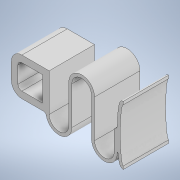
# Autodesk Inventor part: resortePlano0.8mm
Saved by Autodesk Inventor 2021.5 (Build 255421000, 421)
## iProperties
Created: 2024-11-30
Part Number: resortePlano0.8mm
Material: Genérico
Document SubType Name: Modeling
Designer: Joho_
Density: 1 g/cm^3
Appearance: Valor por defecto
Author: Joho_
## iProperties of the stored document _3DPrint.ipt
Created: 2024-11-30
Part Number: _3DPrint
Material: Genérico
Document SubType Name: Modeling
Designer: Joho_
Density: 1 g/cm^3
Appearance: Valor por defecto
Author: Joho_
Autodesk Inventor part; units mm, degrees
ref_plane "YZ Plane" through (0, 0, 0) normal (1, 0, 0) x (0, 1, 0)
ref_plane "XZ Plane" through (0, 0, 0) normal (0, 1, 0) x (-1, 0, 0)
ref_plane "XY Plane" through (0, 0, 0) normal (0, 0, 1) x (1, 0, 0)
sketch "Boceto1" plane through (0, 0, 0) normal (0, 0, 1) x (1, 0, 0)
  line L0 (3, -11.4) -> (3, -5.5)
  line L1 (3, -5.5) -> (-2.2, -5.5)
  arc A0 (-5.5, -2.2) -> (-2.2, -5.5) centre (-2.2, -2.2) ccw
  line L2 (-5.5, -2.2) -> (-5.5, 2.2)
  arc A1 (-2.2, 5.5) -> (-5.5, 2.2) centre (-2.2, 2.2) ccw
  line L3 (-2.2, 5.5) -> (3, 5.5)
  line L4 (3, 5.5) -> (3, 11.4)
  line L5 (3, 3) -> (-2.2, 3)
  arc A2 (-2.2, 3) -> (-3, 2.2) centre (-2.2, 2.2) ccw
  line L6 (-3, 2.2) -> (-3, -2.2)
  arc A3 (-3, -2.2) -> (-2.2, -3) centre (-2.2, -2.2) ccw
  line L7 (-2.2, -3) -> (3, -3)
  line L8 (3, -3) -> (3, 3)
  line L9 (-2.2, 3.25) -> (3.25, 3.25)
  line L10 (3.25, 3.25) -> (3.25, -3.25)
  line L11 (3.25, -3.25) -> (-2.2, -3.25)
  arc A4 (-3.25, -2.2) -> (-2.2, -3.25) centre (-2.2, -2.2) ccw
  line L12 (-3.25, -2.2) -> (-3.25, 2.2)
  arc A5 (-2.2, 3.25) -> (-3.25, 2.2) centre (-2.2, 2.2) ccw
  line L13 (-2.2, 5) -> (5, 5)
  line L14 (5, 5) -> (5, -5)
  line L15 (5, -5) -> (-2.2, -5)
  arc A6 (-5, -2.2) -> (-2.2, -5) centre (-2.2, -2.2) ccw
  line L16 (-5, -2.2) -> (-5, 2.2)
  arc A7 (-2.2, 5) -> (-5, 2.2) centre (-2.2, 2.2) ccw
  line L17 (22.2, 0) -> (23, 0)
  line L18 (10.2, 5) -> (11, 5)
  line L19 (11, 5) -> (11, -5)
  line L20 (11, -5) -> (10.2, -5)
  line L21 (10.2, -5) -> (10.2, 5)
  line L22 (16.2, 5) -> (17, 5)
  line L23 (17, 5) -> (17, -5)
  line L24 (17, -5) -> (16.2, -5)
  line L25 (16.2, -5) -> (16.2, 5)
  line L26 (22.2, 5) -> (23, 5)
  line L27 (23, 0) -> (23, -5)
  line L28 (23, -5) -> (22.2, -5)
  line L29 (22.2, -5) -> (22.2, 0)
  line L30 (17, 5) -> (16.2, 5)
  arc A8 (17, 5) -> (10.2, 5) centre (13.6, 5) ccw
  arc A9 (16.2, 5) -> (11, 5) centre (13.6, 5) ccw
  arc A10 (10.685, 3.25) -> (11, 2.8091) centre (13.6, 5) ccw
  arc A11 (16.2, -5) -> (23, -5) centre (19.6, -5) ccw
  arc A12 (17, -5) -> (22.2, -5) centre (19.6, -5) ccw
  arc A13 (5, -5) -> (10.2, -5) centre (7.6, -5) ccw
  arc A14 (4.2, -5) -> (11, -5) centre (7.6, -5) ccw
  line L31 (24.6, 7) -> (24.6, 7.8)
  ellipse E0 centre (24.6, 0) end of major axis (23.8, 0) minor radius 7 (24.6, 7) -> (24.6, -7) ccw
  line L32 (22.6, 0.6) -> (23.0029, 0.6)
  line L33 (23.8, 0.6) -> (23.8, -0.6)
  line L34 (23.0029, -0.6) -> (22.2, -0.6)
  line L35 (22.2, -0.6) -> (22.2, 0.2)
  line L36 (24.6, -7) -> (24.6, -7.8)
  arc A15 (22.6, 0.6) -> (22.2, 0.2) centre (22.6, 0.2) ccw
  line L37 (23.0029, -0.6) -> (23.8029, -0.6)
  line L38 (23.0029, 0.6) -> (23.8029, 0.6)
  spline S0 degree 5 poles (24.6, 7.8) (24.4963, 7.8002) (24.3925, 7.7852) (24.2917, 7.755) (24.0119, 7.624) (23.7979, 7.3915) (23.7022, 7.2078) (23.5522, 6.8313) (23.4568, 6.4344) (23.4154, 6.2353) (23.3306, 5.7654) (23.267, 5.2931) (23.235, 5.0218) (23.1724, 4.4197) (23.125, 3.8158) (23.1025, 3.4839) (23.0617, 2.7807) (23.0336, 2.077) (23.022, 1.7056) (23.0043, 0.9491) (22.9985, 0.1925) (22.9985, -0.1925) (23.0043, -0.9491) (23.022, -1.7056) (23.0336, -2.077) (23.0617, -2.7807) (23.1025, -3.4839) (23.125, -3.8158) (23.1724, -4.4197) (23.235, -5.0218) (23.267, -5.2931) (23.3306, -5.7654) (23.4154, -6.2353) (23.4568, -6.4344) (23.5522, -6.8313) (23.7022, -7.2078) (23.7979, -7.3915) (24.0119, -7.624) (24.2917, -7.755) (24.3925, -7.7852) (24.4963, -7.8002) (24.6, -7.8) knots 0 0 0 0 0 0 0.030865 0.030865 0.030865 0.090986 0.090986 0.090986 0.15174 0.15174 0.15174 0.232979 0.232979 0.232979 0.332038 0.332038 0.332038 0.442681 0.442681 0.442681 0.557319 0.557319 0.557319 0.667962 0.667962 0.667962 0.767021 0.767021 0.767021 0.84826 0.84826 0.84826 0.909014 0.909014 0.909014 0.969135 0.969135 0.969135 1 1 1 1 1 1
  spline S1 degree 5 poles (24.6, 7.8) (24.4963, 7.8002) (24.3925, 7.7852) (24.2917, 7.755) (24.0119, 7.624) (23.7979, 7.3915) (23.7022, 7.2078) (23.5522, 6.8313) (23.4568, 6.4344) (23.4154, 6.2353) (23.3306, 5.7654) (23.267, 5.2931) (23.235, 5.0218) (23.1724, 4.4197) (23.125, 3.8158) (23.1025, 3.4839) (23.0617, 2.7807) (23.0336, 2.077) (23.022, 1.7056) (23.0043, 0.9491) (22.9985, 0.1925) (22.9985, -0.1925) (23.0043, -0.9491) (23.022, -1.7056) (23.0336, -2.077) (23.0617, -2.7807) (23.1025, -3.4839) (23.125, -3.8158) (23.1724, -4.4197) (23.235, -5.0218) (23.267, -5.2931) (23.3306, -5.7654) (23.4154, -6.2353) (23.4568, -6.4344) (23.5522, -6.8313) (23.7022, -7.2078) (23.7979, -7.3915) (24.0119, -7.624) (24.2917, -7.755) (24.3925, -7.7852) (24.4963, -7.8002) (24.6, -7.8) knots 0 0 0 0 0 0 0.030865 0.030865 0.030865 0.090986 0.090986 0.090986 0.15174 0.15174 0.15174 0.232979 0.232979 0.232979 0.332038 0.332038 0.332038 0.442681 0.442681 0.442681 0.557319 0.557319 0.557319 0.667962 0.667962 0.667962 0.767021 0.767021 0.767021 0.84826 0.84826 0.84826 0.909014 0.909014 0.909014 0.969135 0.969135 0.969135 1 1 1 1 1 1
  point P0 (0, 0)
  point P1 (24.2, 5)
  point P2 (8, 5)
  point P3 (13.2, 5)
  point P4 (19.2, 5)
  point P5 (5, -5)
  point P6 (8, -5)
  point P7 (11, -5)
  point P8 (13.2, -5)
  point P9 (19.2, -5)
  point P10 (23.0029, 0.6)
  point P11 (23.0029, -0.6)
  point P12 (23, -0.6)
  dimension "d1" = 0.25
  dimension "d2" = 2
  dimension "d10" = 0.8
  dimension "d11" = 10
  dimension "d12" = 0.8
  dimension "d13" = 0.8
  constraints: 78 end point, 32 point on circle, 19 centre point, 4 coincident, 3 point on line, 1 horizontal, 14 other
  measures "d1" distance between parallel lines of L5 L9
  measures "d2" distance between parallel lines of L5 L13
  measures "d10" distance of L19.end L20.end
  measures "d11" distance of L18.end L19.end
  measures "d12" distance of L23.end L24.end
  measures "d13" distance of L28.end L27.end
extrude "Extrusión1" add sketch "Boceto1" along normal blind 12 contours L13 L14 L15 A6 L16 A7 | A13 L20 A14 L15 | L21 L18 L19 L20 | A8 L22 A9 L18 | L23 L24 L25 L22 | A12 L28 A11 L24 | L29 L34 L27 L28 | L29 L17 L27 L34 | L27 S0 L34 | L35 A15 L32 S0 L17 | S0 L38 L33 L37 | L37 E0 L36 S0 | S0 L31 E0 L38 | L33 E0 L37 | L38 E0 L33
fillet "Empalme1" radius 0.8 2 edges at (4.2, -5, 6) (23.0029, 0.6, 6)
fillet "Empalme1" radius 0.1 2 edges at (23.0029, -0.6, 6) (23, -0.6, 6)
